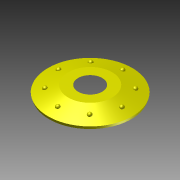
# Autodesk Inventor part: Suction Cup Part 2 1764
Saved by Autodesk Inventor 2011 (Build 150239000, 239)
## iProperties
Created: 2010-02-08
Part Number: Suction Cup Part 2 1764
Document SubType Name: Modeling
Designer: clee1
Density: 1 g/cm^3
Author: clee1
Autodesk Inventor part; units mm, degrees
ref_plane "XZ Plane" through (0, 0, 0) normal (0, 1, 0) x (-1, 0, 0)
ref_plane "XY Plane" through (0, 0, 0) normal (0, 0, 1) x (1, 0, 0)
sketch "Sketch1" plane through (0, 0, 0) normal (0, 0, 1) x (1, 0, 0)
  line L0 (14.769106, 15.753687) -> (-2.838656, 10.201981)
  line L1 (8.727218, 15.753687) -> (-3.384987, 11.934724)
  line L2 (-2.838656, 10.201981) -> (-3.384987, 11.934724)
  line L3 (14.769106, 15.753687) -> (8.727218, 15.753687)
  line L4 (22.015013, 28.238546) -> (22.015013, -0.513428)
  point P0 (0, 0)
  point P1 (0, 0)
  dimension "d0" = 25.4
  constraints: 10 end point, 1 perpendicular
  measures "d0" distance from line of L2.end L4
revolve "Revolution1" add sketch "Sketch1" angle 360 about axis through (22.015013, 28.238546, 0) along (0, -1, 0)
ref_plane "Work Plane1" through (22.225, 0, 0) normal (1, 0, 0) x (0, 1, 0)
sketch "Sketch2" plane through (22.225, 0, 0) normal (1, 0, 0) x (0, 1, 0)
  line L0 (11.934724, -25.4) -> (15.753687, -13.287795)
  line L1 (15.753687, -13.287795) -> (15.753687, 13.287795)
  line L2 (11.934724, -25.4) -> (11.934724, 25.4)
  line L3 (15.753687, -13.287795) -> (19.177332, -14.367266)
  line L4 (11.934724, -25.4) -> (15.348905, -26.476487)
  line L5 (13.844205, -19.343897) -> (22.039279, -21.927794)
  arc A0 (13.462309, -20.555118) -> (15.055426, -19.725794) centre (13.844205, -19.343897) ccw
  line L6 (13.844205, -19.343897) -> (13.462309, -20.555118)
  line L7 (15.055426, -19.725794) -> (13.844205, -19.343897)
  point P0 (0, 0)
  dimension "d3" = 0
  dimension "d6" = 6.35
  dimension "d7" = 6.35
  constraints: 10 end point, 2 parallel, 2 perpendicular, 2 point on circle, 2 point on line, 1 centre point, 1 collinear
  measures "d3" distance from line of L0 L5.start
  measures "d6" distance from line of L3 L5.start
  measures "d7" distance from line of L4 L5.start
revolve "Revolution2" add sketch "Sketch2" angle 360 about axis through (22.225, 13.844205, -19.343897) along (0, 0.953717, -0.3007058)
pattern_circular "Circular Pattern1" count 8 over 360 about axis through (22.015013, 13.844205, 0) along (0, 1, 0) of "Revolution2"
body "Solid1"
